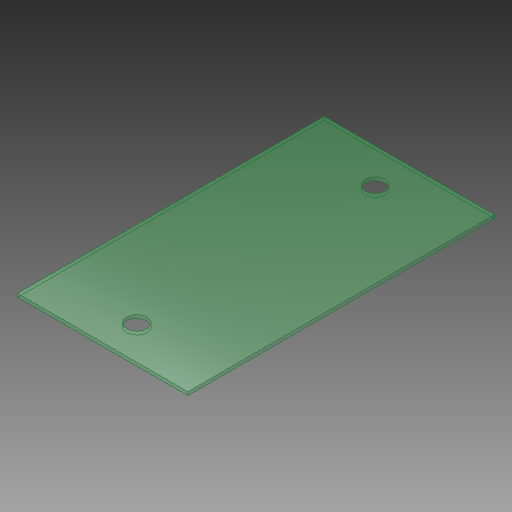
# Autodesk Inventor part: sb_bottom
Saved by Autodesk Inventor 2018.1 (Build 221171000, 171)
## iProperties
Created: 2017-08-17
Part Number: sb_bottom
Material: PVC-Piping
Document SubType Name: Modeling
Designer: Tom
Density: 1.4 g/cm^3
Appearance: Clear - Green 1
Author: Tom
Autodesk Inventor part; units mm, degrees
ref_plane "YZ Plane" through (0, 0, 0) normal (1, 0, 0) x (0, 1, 0)
ref_plane "XZ Plane" through (0, 0, 0) normal (0, 1, 0) x (-1, 0, 0)
ref_plane "XY Plane" through (0, 0, 0) normal (0, 0, 1) x (1, 0, 0)
sketch "Sketch1" plane through (0, 0, 0) normal (0, 1, 0) x (-1, 0, 0)
  line L0 (125, 225) -> (-125, 225)
  line L1 (-125, 225) -> (-125, -225)
  line L2 (-125, -225) -> (125, -225)
  line L3 (125, -225) -> (125, 225)
  line L4 (125, 225) -> (-125, -225) construction
  line L5 (-125, 225) -> (125, -225) construction
  point P0 (0, 0)
  dimension "d0" = 250
  dimension "d1" = 450
  constraints: 12 end point, 2 midpoint, 2 parallel, 1 horizontal, 1 perpendicular
  measures "d0" distance of L2.end L1.end
  measures "d1" distance of L1.end L0.end
extrude "Extrusion1" add sketch "Sketch1" along normal blind 5
sketch "Sketch2" plane through (0, 0, 0) normal (0, -1, 0) x (1, 0, 0)
  circle A0 centre (0, 175) radius 15
  line L0 (-125, 225) -> (125, 225) projected
  line L1 (-125, 0) -> (125, 0) construction
  line L2 (125, 225) -> (125, -225) construction
  circle A1 centre (0, -175) radius 15
  point P0 (0, 0)
  dimension "d4" = 30
  dimension "d5" = 50
  constraints: 2 centre point, 2 end point, 1 midpoint, 1 symmetric about line, 1 other
  measures "d4" diameter of A0
  measures "d5" distance from line of L0 A0.centre
extrude "Extrusion2" cut sketch "Sketch2" against normal blind 5
equation "\"d0\" = boxl"
equation "\"d1\" = boxw"
equation "\"d2\" = pvct"
equation "\"d6\" = pvct"
equation "\"solhole\" = 3"
equation "\"solholespacing\" = 16"
equation "\"ssolw\" = 63"
equation "\"bsoll\" = 126"
equation "\"bsolw\" = 91"
equation "\"bsolh\" = 126"
equation "\"tapl\" = 31"
equation "\"tl\" = 32"
equation "\"eloboww\" = 25"
equation "\"pvct\" = 5"
equation "\"boxw\" = 450"
equation "\"boxl\" = 250"
equation "\"boxh\" = 258"
equation "\"supporth\" = 15"
equation "\"play\" = 0.5"
equation "\"arw\" = 54"
equation "\"arl\" = 102"
equation "\"psuh\" = 85"
equation "\"screenw\" = 197"
equation "\"screenl\" = 115"
equation "\"pcbw\" = 76"
equation "\"pcbl\" = 86"
equation "\"pcbh\" = 46"
equation "\"seph\" = 105"
equation "\"diapowerouter\" = 25"
equation "\"dialoadouter\" = 25"
equation "\"diaetape\" = 25"
equation "\"distpumps\" = 75"
equation "\"diaph\" = 32"
equation "\"diaetapeouter\" = 36"
equation "\"diaphouter\" = 48"
equation "\"diaload\" = 16"
equation "\"distbubblewater\" = 82"
equation "\"diapower\" = 16"
equation "\"pumpinner\" = 16"
equation "\"airoutouter\" = 39"
equation "\"airinouter\" = 39"
equation "\"waterouter\" = 39"
equation "\"airininner\" = 28"
equation "\"waterinner\" = 28"
equation "\"airoutinner\" = 28"
equation "\"pumpouter\" = 25"
body "Solid1"
